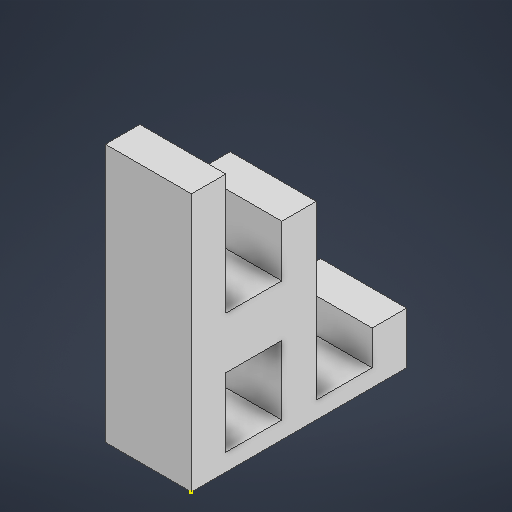
# Autodesk Inventor part: Part3
Saved by Autodesk Inventor 2026 (Build 300175000, 175)
## iProperties
Created: 2025-05-05
Part Number: Part3
Material: Generic
Document SubType Name: Sheet Metal
Designer: 18438
Density: 1 g/cm^3
Sheet Metal Rule: Default_mm
Appearance: Default
Author: 18438
Autodesk Inventor part; units mm, degrees
ref_plane "YZ Plane" through (0, 0, 0) normal (1, 0, 0) x (0, 1, 0)
ref_plane "XZ Plane" through (0, 0, 0) normal (0, 1, 0) x (-1, 0, 0)
ref_plane "XY Plane" through (0, 0, 0) normal (0, 0, 1) x (1, 0, 0)
sketch "Sketch1" plane through (0, 0, 0) normal (0, 1, 0) x (-1, 0, 0)
  line L0 (0, 0) -> (50, 0)
  line L1 (50, 0) -> (50, -125)
  line L2 (50, -125) -> (0, -125)
  line L3 (0, -125) -> (0, 0)
  dimension "d0" = 50
  dimension "d1" = 125
  constraints: 8 end point, 2 parallel, 1 horizontal, 1 perpendicular
  measures "d0" distance of L1.end L2.end
  measures "d1" distance of L0.end L1.end
extrude "Extrusion1" add sketch "Sketch1" along normal blind 10
sketch "Sketch2" plane through (0, 10, 0) normal (0, 1, 0) x (1, 0, 0)
  line L0 (-50, 125) -> (-50, 0) projected
  line L1 (0, 0) -> (0, 125) projected
  line L2 (-50, 0) -> (0, 0)
  line L3 (0, 0) -> (0, 20)
  line L4 (0, 20) -> (-50, 20)
  line L5 (-50, 20) -> (-50, 0)
  line L6 (0, 125) -> (-50, 125) projected
  line L7 (-50, 125) -> (0, 125)
  line L8 (0, 125) -> (0, 105)
  line L9 (0, 105) -> (-50, 105)
  line L10 (-50, 105) -> (-50, 125)
  line L11 (-50, 62.5) -> (0, 62.5)
  line L12 (0, 62.5) -> (0, 72.5)
  line L13 (0, 72.5) -> (-50, 72.5)
  line L14 (-50, 72.5) -> (-50, 62.5)
  line L15 (-50, 62.5) -> (0, 62.5)
  line L16 (0, 62.5) -> (0, 52.5)
  line L17 (0, 52.5) -> (-50, 52.5)
  line L18 (-50, 52.5) -> (-50, 62.5)
  dimension "d4" = 20
  dimension "d5" = 20
  dimension "d6" = 10
  dimension "d7" = 10
  constraints: 32 end point, 8 parallel, 4 horizontal, 4 perpendicular, 4 point on line, 1 midpoint
  measures "d4" distance of L3.end L2.end
  measures "d5" distance of L7.end L8.end
  measures "d6" distance of L12.end L11.end
  measures "d7" distance of L15.end L16.end
extrude "Extrusion2" add sketch "Sketch2" along normal blind 20 contours L6 L1 L9 L0 | L13 L1 L11 L0 | L11 L1 L17 L0 | L4 L1 L2 L0
sketch "Sketch3" plane through (0, 30, 0) normal (0, 1, 0) x (1, 0, 0)
  line L0 (0, 20) -> (0, 52.5) projected
  line L1 (-50, 0) -> (0, 0)
  line L2 (0, 0) -> (0, 20)
  line L3 (0, 20) -> (-50, 20)
  line L4 (-50, 20) -> (-50, 0)
  line L5 (-50, 52.5) -> (0, 52.5) projected
  line L6 (0, 72.5) -> (-50, 72.5) projected
  line L7 (-50, 52.5) -> (0, 52.5)
  line L8 (0, 52.5) -> (0, 72.5)
  line L9 (0, 72.5) -> (-50, 72.5)
  line L10 (-50, 72.5) -> (-50, 52.5)
  constraints: 16 end point, 4 parallel, 2 horizontal, 2 perpendicular
extrude "Extrusion3" add sketch "Sketch3" along normal blind 100
sketch "Sketch4" plane through (0, 10, -20) normal (0, 0, -1) x (-1, 0, 0)
  line L0 (0, 0) -> (0, 120) projected
  line L1 (50, 0) -> (50, 120) projected
  line L2 (0, 120) -> (50, 120)
  line L3 (50, 120) -> (50, 100)
  line L4 (50, 100) -> (0, 100)
  line L5 (0, 100) -> (0, 120)
  line L6 (50, 100) -> (0, 100)
  line L7 (0, 100) -> (0, 70)
  line L8 (0, 70) -> (50, 70)
  line L9 (50, 70) -> (50, 100)
  line L10 (0, 70) -> (50, 70)
  line L11 (50, 70) -> (50, 40)
  line L12 (50, 40) -> (0, 40)
  line L13 (0, 40) -> (0, 70)
  point P0 (0, -10)
  dimension "d12" = 20
  dimension "d13" = 30
  dimension "d14" = 30
  constraints: 24 end point, 6 parallel, 3 horizontal, 3 perpendicular, 3 point on line
  measures "d12" distance of L2.end L3.end
  measures "d13" distance of L7.end L6.end
  measures "d14" distance of L10.end L11.end
extrude "Extrusion4" add sketch "Sketch4" along normal blind 40 contours L0 L8 L1 L12
sketch "Sketch5" plane through (0, 130, 0) normal (0, 1, 0) x (1, 0, 0)
  line L0 (-50, 105) -> (-50, 72.5) projected
  line L1 (0, 52.5) -> (-50, 52.5)
  line L2 (-50, 52.5) -> (-50, 72.5)
  line L3 (-50, 72.5) -> (0, 72.5)
  line L4 (0, 72.5) -> (0, 52.5)
  point P0 (0, 0)
  constraints: 8 end point, 2 parallel, 1 horizontal, 1 perpendicular
extrude "Extrusion5" cut sketch "Sketch5" against normal blind 20
sketch "Sketch6" plane through (0, 0, 0) normal (1, 0, 0) x (0, 0, -1)
  point P0 (0, 0)
sketch "Sketch7" plane through (0, 130, 0) normal (0, 1, 0) x (1, 0, 0)
  line L0 (-50, 0) -> (0, 0) projected
  line L1 (-50, 20) -> (0, 20) projected
  line L2 (0, 0) -> (-50, 0)
  line L3 (-50, 0) -> (-50, 20)
  line L4 (-50, 20) -> (0, 20)
  line L5 (0, 20) -> (0, 0)
  constraints: 8 end point, 2 parallel, 1 horizontal, 1 perpendicular
extrude "Extrusion6" add sketch "Sketch7" along normal blind 20
equation "\"BendRadius\" = Thickness"
equation "\"BendReliefWidth\" = Thickness"
equation "\"BendReliefDepth\" = 0.5 * Thickness"
equation "\"CornerReliefSize\" = 4 * Thickness"
equation "\"MinimumRemnant\" = 2 * Thickness"
equation "\"TransitionRadius\" = BendRadius"
equation "\"JacobiRadiusSize\" = BendRadius"
equation "\"GapSize\" = Thickness"
equation "\"Thickness\" = 0.5"
body "Solid1"
